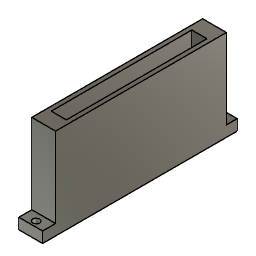
batteryholder (Autodesk Fusion 360 design; units mm, degrees)
part number: 2025-05-06-22-04-36-010
Autodesk Fusion 360 part; units mm, degrees
sketch "Sketch1" plane through (0, 0, 0) normal (0, 1, 0) x (1, 0, 0)
  line L0 (2, 0) -> (40, 0)
  line L1 (40, 0) -> (40, -61)
  line L2 (40, -61) -> (2, -61)
  line L3 (2, -61) -> (2, 0)
  dimension "d1" = 38
  dimension "d2" = 61
  constraint horizontal L0
  constraint vertical L1
  constraint horizontal L2
  constraint vertical L3
  measures "d1" distance of L0.start L0.end
  measures "d2" distance of L0.start L2.end
sketch "Sketch2" plane through (0, 0, 61) normal (0, 0, 1) x (-1, 0, 0)
  line L0 (-2, 0) -> (-40, 0)
  line L1 (-40, 0) -> (-40, -8)
  line L2 (-40, -8) -> (-2, -8)
  line L3 (-2, -8) -> (-2, 0)
  line L4 (-2, -7) -> (-40, -7)
  line L5 (-40, -1) -> (-39.6486, -1)
  line L6 (-39.6486, -1) -> (-2, -1)
  line L7 (-2, -1) -> (-3, -1)
  line L8 (-2, -7) -> (-3, -7)
  line L9 (-2, -7) -> (-3, -7)
  line L10 (-40, -7) -> (-39, -7)
  line L11 (-40, -1) -> (-39, -1)
  line L12 (-40, -1) -> (-39, -1)
  line L13 (-2, -7) -> (-2.5, -7)
  line L14 (-40, -7) -> (-39.5, -7)
  line L15 (-40, -1) -> (-39.5, -1)
  line L16 (-2, -1) -> (-2.5, -1)
  line L17 (-2.5, -8) -> (-2.5, 0)
  line L18 (-39.5, -8) -> (-39.5, 0)
  line L19 (-2, -8) -> (-1.5, -8)
  line L20 (-1.5, -8) -> (-1.5, 0)
  line L21 (-1.5, 0) -> (-2, 0)
  line L22 (-2, 0) -> (-2, -8)
  line L23 (-40, -8) -> (-40.5, -8)
  line L24 (-40.5, -8) -> (-40.5, 0)
  line L25 (-40.5, 0) -> (-40, 0)
  line L26 (-40, 0) -> (-40, -8)
  dimension "d5" = 0.5
  dimension "d6" = 0.5
  dimension "d7" = 0.5
  dimension "d8" = 0.5
  dimension "d9" = 0.5
  dimension "d10" = 8
  dimension "d11" = 0.5
  constraint coincident L3 L4.start
  constraint coincident L1 L4.end
  constraint perpendicular L1 L4
  constraint coincident L1 L5.start
  constraint perpendicular L1 L5
  constraint coincident L3 L6.end
  constraint perpendicular L3 L6
  constraint coincident L6 L7.end
  constraint perpendicular L3 L7
  constraint coincident L4 L8.end
  constraint coincident L4 L10.end
  constraint coincident L6 L11.end
  constraint perpendicular L1 L11
  constraint perpendicular L3 L13
  constraint perpendicular L1 L14
  constraint parallel L11 L15
  constraint perpendicular L3 L16
  constraint coincident L2 L17.start
  constraint coincident L0 L17.end
  constraint perpendicular L0 L17
  constraint coincident L2 L18.start
  constraint coincident L0 L18.end
  constraint perpendicular L0 L18
  constraint horizontal L19
  constraint vertical L20
  constraint horizontal L21
  constraint vertical L22
  constraint coincident L2.end L3.start
  constraint horizontal L23
  constraint vertical L24
  constraint horizontal L25
  constraint vertical L26
  constraint coincident L1.end L2.start
  measures "d5" distance of L4.start L13.end
  measures "d6" distance of L4.end L14.end
  measures "d7" distance of L5.start L15.end
  measures "d8" distance of L6.end L16.end
  measures "d9" distance of L2.end L19.end
  measures "d10" distance of L2.end L0.start
  measures "d11" distance of L1.end L23.end
sketch "Sketch3" plane through (0, 0, 61) normal (0, 0, 1) x (-1, 0, 0)
sketch "Sketch4" plane through (0, 0, 0) normal (1, 0, 0) x (0, 1, 0)
  line L0 (5, 0) -> (41.5, 0)
  line L1 (41.5, 0) -> (41.5, 59.5)
  line L2 (41.5, 59.5) -> (5, 59.5)
  line L3 (5, 59.5) -> (5, 0)
  dimension "d24" = 36.5
  dimension "d25" = 59.5
  constraint horizontal L0
  constraint vertical L1
  constraint horizontal L2
  constraint vertical L3
  measures "d24" distance of L0.start L0.end
  measures "d25" distance of L0.start L2.end
extrude "Extrude3" add sketch "Sketch4" along normal blind 5 makes body 1
sketch "Sketch5" plane through (5, 0, 0) normal (1, 0, 0) x (0, 1, 0)
  line L0 (5, 59.5) -> (5, 0)
  line L1 (5, 0) -> (41.5, 0)
  line L2 (41.5, 0) -> (41.5, 59.5)
  line L3 (41.5, 59.5) -> (5, 59.5)
  line L4 (-5, -5) -> (50, -5)
  line L5 (50, -5) -> (50, 60)
  line L6 (50, 60) -> (-5, 60)
  line L7 (-5, 60) -> (-5, -5)
  constraint horizontal L4
  constraint vertical L5
  constraint horizontal L6
  constraint vertical L7
extrude "Extrude4" add sketch "Sketch5" along normal blind 7 separate body contours L0 L1 L2 L3 | L4 L5 L6 L7 makes body 2
sketch "Sketch6" plane through (0, 41.5, 0) normal (0, 1, 0) x (-1, 0, 0)
  line L0 (0, 0) -> (0, 59.5)
  line L1 (0, 59.5) -> (-5, 59.5)
  line L2 (-5, 59.5) -> (-5, 0)
  line L3 (-5, 0) -> (0, 0)
  line L4 (-5, 60) -> (0, 60)
  line L5 (0, 60) -> (0, -5)
  line L6 (0, -5) -> (-5, -5)
  line L7 (-5, -5) -> (-5, 60)
  constraint horizontal L4
  constraint vertical L5
  constraint horizontal L6
  constraint vertical L7
extrude "Extrude5" add sketch "Sketch6" along normal blind 8.5 contours L0 L1 L2 L3 L5 L7 | L3 L5 L6 L7 bodies 1 2
sketch "Sketch7" plane through (5, 0, 0) normal (-1, 0, 0) x (0, -1, 0)
  line L0 (-41.5, 0) -> (-41.5, -5)
  line L1 (-41.5, -5) -> (5, -5)
  line L2 (5, -5) -> (5, 60)
  line L3 (5, 60) -> (-50, 60)
  line L4 (-50, 60) -> (-50, 59.5)
  line L5 (-50, 59.5) -> (-5, 59.5)
  line L6 (-5, 59.5) -> (-5, 0)
  line L7 (-5, 0) -> (-41.5, 0)
  line L8 (-5, 60) -> (5, 60)
  line L9 (5, 60) -> (5, -5)
  line L10 (5, -5) -> (-5, -5)
  line L11 (-5, -5) -> (-5, 60)
  line L12 (-41.5, -5) -> (-5, -5)
  line L13 (-5, -5) -> (-5, 0)
  line L14 (-5, 0) -> (-41.5, 0)
  line L15 (-41.5, 0) -> (-41.5, -5)
  constraint horizontal L8
  constraint vertical L9
  constraint horizontal L10
  constraint vertical L11
  constraint coincident L1.end L2.start
  constraint coincident L3 L8.start
  constraint horizontal L12
  constraint vertical L13
  constraint horizontal L14
  constraint vertical L15
  constraint coincident L6.end L7.start
  constraint coincident L0.end L1.start
extrude "Extrude6" add sketch "Sketch7" along normal blind 5 contours L0 L1 L7 L11 L12 L13 L14 L15 | L1 L2 L3 L6 L8 L9 L10 L11 L13 bodies 1
sketch "Sketch8" plane through (0, 0, 0) normal (-1, 0, 0) x (0, -1, 0)
  line L0 (-5, 59.5) -> (-50, 59.5)
  line L1 (-50, 59.5) -> (-50, -5)
  line L2 (-50, -5) -> (5, -5)
  line L3 (5, -5) -> (5, 60)
  line L4 (5, 60) -> (-5, 60)
  line L5 (-5, 60) -> (-5, 59.5)
  line L6 (5, 60) -> (-50, 60)
  line L7 (-50, 60) -> (-50, -5)
  line L8 (-50, -5) -> (5, -5)
  line L9 (5, -5) -> (5, 60)
  constraint horizontal L6
  constraint vertical L7
  constraint horizontal L8
  constraint vertical L9
  constraint coincident L1.end L2.start
  constraint coincident L3.end L4.start
extrude "Extrude7" add sketch "Sketch8" along normal blind 7 contours L0 L1 L2 L3 L4 L5 L6 L7 L8 L9 bodies 1
sketch "Sketch9" plane through (0, 0, 59.5) normal (0, 0, 1) x (-1, 0, 0)
  line L0 (7, -5) -> (-5, -5)
  line L1 (-5, -5) -> (-5, -50)
  line L2 (-5, -50) -> (7, -50)
  line L3 (7, -50) -> (7, -5)
  line L4 (-5, -5) -> (0, -5)
  line L5 (0, -5) -> (0, -41.5)
  line L6 (0, -41.5) -> (-5, -41.5)
  line L7 (-5, -41.5) -> (-5, -5)
  dimension "d38" = 5
  dimension "d39" = 36.5
  constraint horizontal L4
  constraint vertical L5
  constraint horizontal L6
  constraint vertical L7
  constraint coincident L0.end L1.start
  measures "d38" distance of L0.end L4.end
  measures "d39" distance of L0.end L6.end
extrude "Extrude8" add sketch "Sketch9" along normal blind 0.5 contours L0 L1 L2 L3 L5 L6 bodies 1
extrude "Extrude9" cut 1 faces at (1.6667, 29.3333, 59.5) along direction (0, 0, -1) blind 59.5 on bodies 1 bodies 1
sketch "Sketch10" plane through (0, 0, 60) normal (0, 0, 1) x (-1, 0, 0)
  line L0 (7, -50) -> (7, 5)
  line L1 (7, 5) -> (-12, 5)
  line L2 (-12, 5) -> (-12, -50)
  line L3 (-12, -50) -> (7, -50)
  line L4 (0, -5) -> (0, -41.5)
  line L5 (0, -41.5) -> (-5, -41.5)
  line L6 (-5, -41.5) -> (-5, -5)
  line L7 (-5, -5) -> (0, -5)
  line L8 (-6, -4) -> (1, -4)
  line L9 (1, -4) -> (1, -43)
  line L10 (1, -43) -> (-6, -43)
  line L11 (-6, -43) -> (-6, -4)
  constraint horizontal L8
  constraint vertical L9
  constraint horizontal L10
  constraint vertical L11
extrude "Extrude10" cut sketch "Sketch10" against normal blind 59.5 contours L8 L9 L10 L11 bodies 1
sketch "Sketch11" plane through (0, 50, 0) normal (0, 1, 0) x (-1, 0, 0)
  line L0 (7, 60) -> (-12, 60)
  line L1 (-12, 60) -> (-12, -5)
  line L2 (-12, -5) -> (7, -5)
  line L3 (7, -5) -> (7, 60)
  line L4 (-12, -5) -> (7, -5)
  line L5 (7, -5) -> (7, 5)
  line L6 (7, 5) -> (-12, 5)
  line L7 (-12, 5) -> (-12, -5)
  dimension "d46" = 19
  dimension "d47" = 10
  constraint horizontal L4
  constraint vertical L5
  constraint horizontal L6
  constraint vertical L7
  constraint coincident L1.end L2.start
  measures "d46" distance of L1.end L2.end
  measures "d47" distance of L1.end L6.end
extrude "Extrude11" add sketch "Sketch11" along normal blind 6 contours L1 L2 L3 L4 L5 L6 L7 bodies 1
sketch "Sketch12" plane through (0, 0, 5) normal (0, 0, 1) x (-1, 0, 0)
  line L0 (7, -50) -> (-12, -50)
  line L1 (-12, -50) -> (-12, -56)
  line L2 (-12, -56) -> (7, -56)
  line L3 (7, -56) -> (7, -50)
  circle A0 centre (-2.5, -53) radius 1.5
  dimension "d50" = 3
  measures "d50" diameter of A0
extrude "Extrude12" cut sketch "Sketch12" against normal blind 13 contours A0 bodies 1
sketch "Sketch13" plane through (0, -5, 0) normal (0, -1, 0) x (1, 0, 0)
  line L0 (-7, -5) -> (12, -5)
  line L1 (12, -5) -> (12, 60)
  line L2 (12, 60) -> (-7, 60)
  line L3 (-7, 60) -> (-7, -5)
  line L4 (-7, -5) -> (12, -5)
  line L5 (12, -5) -> (12, 5)
  line L6 (12, 5) -> (-7, 5)
  line L7 (-7, 5) -> (-7, -5)
  dimension "d53" = 10
  constraint horizontal L4
  constraint vertical L5
  constraint horizontal L6
  constraint vertical L7
  constraint coincident L0.start L3.end
  measures "d53" distance of L0.start L6.end
extrude "Extrude13" add sketch "Sketch13" along normal blind 6 contours L0 L1 L3 L4 L5 L6 L7 bodies 1
sketch "Sketch14" plane through (0, 0, 5) normal (0, 0, 1) x (-1, 0, 0)
  line L0 (-12, 5) -> (7, 5)
  line L1 (7, 5) -> (7, 11)
  line L2 (7, 11) -> (-12, 11)
  line L3 (-12, 11) -> (-12, 5)
  circle A0 centre (-2.5, 8) radius 1.5
  dimension "d56" = 3
  measures "d56" diameter of A0
extrude "Extrude14" cut sketch "Sketch14" against normal blind 17 contours A0 bodies 1
extrude "Extrude15" add 1 faces at (5.6667, 56, 1.6667) along direction (0, 1, 0) blind 25 on bodies 1 bodies 1
extrude "Extrude16" add 1 faces at (3.3333, 50, 23.3333) along direction (0, 1, 0) blind 26 on bodies 1 bodies 1
extrude "Extrude17" cut 1 faces at (1.3333, 43, 20.3333) along direction (0, 1, 0) blind 26 on bodies 1 bodies 1
extrude "Extrude18" add 1 faces at (1.6667, 29.3333, 0) along direction (0, 0, 1) blind 0.5 on bodies 1 bodies 1
extrude "Extrude19" add sketch "Sketch12" against normal blind 10 contours A0 bodies 1
extrude "Extrude20" cut 1 faces at (2.6827, 52.5346, 5) along direction (0, 0, -1) blind 4.5 on bodies 1 bodies 1
extrude "Extrude21" cut 1 faces at (1.6667, -5, 23.3333) along direction (0, 1, 0) blind 2 on bodies 1 bodies 1
extrude "Extrude22" add 1 faces at (-0.6667, -11, 1.6667) along direction (0, 1, 0) blind 8 on bodies 1 bodies 1
extrude "Extrude23" cut 1 faces at (-0.6667, -11, 1.6667) along direction (0, 1, 0) blind 2 on bodies 1 bodies 1
extrude "Extrude24" cut 2 faces at (10, 25.6667, 60) (-2.6667, -0.6667, 60) along direction (0, 0, -1) blind 18 on bodies 1 bodies 1
extrude "Extrude25" add 1 faces at (5.6667, 21, -5) along direction (0, 0, -1) blind 5 on bodies 1 bodies 1
extrude "Extrude26" cut 1 faces at (5.6667, 21, -10) along direction (0, 0, 1) blind 10 on bodies 1 bodies 1
sketch "Sketch15" plane through (0, 0, 5) normal (0, 0, 1) x (-1, 0, 0)
  line L0 (7, 9) -> (-12, 9)
  line L1 (-12, 9) -> (-12, 3)
  line L2 (7, 3) -> (7, 9)
  line L3 (7, 9) -> (-12, 9)
  line L4 (-2.5, 9) -> (-2.5, 6.5)
  circle A0 centre (-2.5, 6.5) radius 1.6
  line L5 (7, 9) -> (7, -81)
  line L6 (7, -81) -> (7, -36)
  line L7 (7, -36) -> (-12, -36)
  circle A1 centre (-2.5, -78.5) radius 1.6
  line L8 (-12, 3) -> (7, 3)
  dimension "d85" = 2.5
  dimension "d86" = 3.2
  constraint coincident L0.start L2.end
  constraint coincident L0.end L1.start
  constraint midpoint L3 L4.start
  constraint perpendicular L3 L4
  constraint coincident L4.end A0.centre
  constraint perpendicular L0 L5
  constraint midpoint L5 L6.end
  constraint perpendicular L5 L7
  constraint symmetric A0 L7 A1
  measures "d85" distance of L4.start L4.end
  measures "d86" diameter of A0
extrude "Extrude27" cut sketch "Sketch15" against normal blind 10 contours A0 | A1 bodies 1
sketch "Sketch16" plane through (0, 69, 0) normal (0, -1, 0) x (1, 0, 0)
  line L0 (6, 42) -> (-1, 42)
  line L1 (-1, 42) -> (-1, 0.5)
  line L2 (-1, 0.5) -> (6, 0.5)
  line L3 (6, 0.5) -> (6, 42)
  line L4 (6, 0.5) -> (-1, 0.5)
  line L5 (-1, 0.5) -> (-1, 3.5)
  line L6 (-1, 3.5) -> (6, 3.5)
  line L7 (6, 3.5) -> (6, 0.5)
  line L8 (-1, 3.5) -> (6, 3.5)
  line L9 (6, 3.5) -> (6, 4.5)
  line L10 (6, 4.5) -> (-1, 4.5)
  line L11 (-1, 4.5) -> (-1, 3.5)
  line L12 (6, 4.5) -> (-1, 4.5)
  line L13 (-1, 4.5) -> (-1, 5.5)
  line L14 (-1, 5.5) -> (6, 5.5)
  line L15 (6, 5.5) -> (6, 4.5)
  line L16 (-1, 5.5) -> (6, 5.5)
  line L17 (6, 5.5) -> (6, 15.5)
  line L18 (6, 15.5) -> (-1, 15.5)
  line L19 (-1, 15.5) -> (-1, 5.5)
  dimension "d89" = 3
  dimension "d90" = 1
  dimension "d91" = 1
  dimension "d92" = 7
  dimension "d93" = 10
  constraint horizontal L4
  constraint vertical L5
  constraint horizontal L6
  constraint vertical L7
  constraint coincident L2.end L3.start
  constraint horizontal L8
  constraint vertical L9
  constraint horizontal L10
  constraint vertical L11
  constraint horizontal L12
  constraint vertical L13
  constraint horizontal L14
  constraint vertical L15
  constraint horizontal L16
  constraint vertical L17
  constraint horizontal L18
  constraint vertical L19
  measures "d89" distance of L2.end L6.end
  measures "d90" distance of L5.end L10.end
  measures "d91" distance of L9.end L14.end
  measures "d92" distance of L13.end L14.end
  measures "d93" distance of L13.end L18.end
extrude "Extrude28" cut sketch "Sketch16" against normal blind 13 contours L1 L3 L14 L16 L17 L18 L19 bodies 1
extrude "Extrude29" cut 1 faces at (12, 23.3333, 29.6667) along direction (-1, 0, 0) blind 4 on bodies 1 bodies 1
extrude "Extrude30" cut 1 faces at (-7, 26, 17.3333) along direction (1, 0, 0) blind 4 on bodies 1 bodies 1
equation "d59 = 64 mm - 39 mm"
equation "d61 = 65 mm - 39 mm"
equation "d63 = -65 mm + 39 mm"
equation "d77 = -55 mm + 37 mm"
